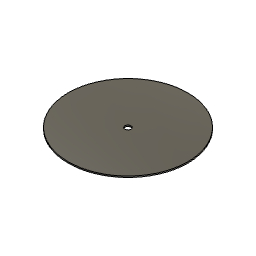
dreidel_prototype (Autodesk Fusion 360 design; units mm, degrees)
Autodesk Fusion 360 part; units mm, degrees
sketch "Sketch1" plane through (0, 0, 0) normal (0, 0, 1) x (1, 0, 0)
  circle A0 centre (0, 0) radius 50
  dimension "d1" = 100
  constraint coincident A0.centre origin
  measures "d1" diameter of A0
extrude "Extrude1" add sketch "Sketch1" along normal blind 1
hole "Hole1" at (0.0785, -0.146, 1) direction (0, 0, -1) diameter 5 depth 1 tip angle 180
